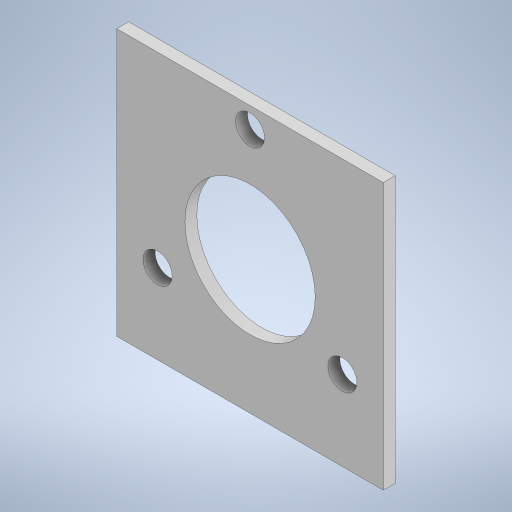
# Autodesk Inventor part: mount_v06
Saved by Autodesk Inventor 2024 (Build 280153000, 153)
## iProperties
Created: 2025-07-16
Part Number: mount_v06
Material: Generic
Document SubType Name: Modeling
Designer: Akramilab
Density: 1 g/cm^3
Appearance: Default
Author: Akramilab
Autodesk Inventor part; units mm, degrees
ref_plane "YZ Plane" through (0, 0, 0) normal (1, 0, 0) x (0, 1, 0)
ref_plane "XZ Plane" through (0, 0, 0) normal (0, 1, 0) x (-1, 0, 0)
ref_plane "XY Plane" through (0, 0, 0) normal (0, 0, 1) x (1, 0, 0)
sketch "Sketch1" plane through (0, 0, 0) normal (0, 0, 1) x (1, 0, 0)
  line L0 (-22.5, -22.5) -> (22.5, -22.5)
  line L1 (22.5, -22.5) -> (22.5, 22.5)
  line L2 (22.5, 22.5) -> (-22.5, 22.5)
  line L3 (-22.5, 22.5) -> (-22.5, -22.5)
  line L4 (-22.5, -22.5) -> (22.5, 22.5) construction
  line L5 (22.5, -22.5) -> (-22.5, 22.5) construction
  circle A0 centre (0, 0) radius 11
  line L6 (0, 0) -> (0, 19)
  line L7 (0, 0) -> (15.6, -9.0067)
  line L8 (0, 0) -> (-15.6, -9.0067)
  circle A1 centre (0, 19) radius 2.45
  circle A2 centre (15.6, -9.0067) radius 2.45
  circle A3 centre (-15.6, -9.0067) radius 2.45
  point P0 (22.5, -11.0947)
  point P1 (-22.5, -11.0947)
  dimension "d0" = 45
  dimension "d1" = 45
  dimension "d2" = 22
  dimension "d3" = 19
  dimension "d4" = 15.6
  dimension "d5" = 120
  dimension "d6" = 15.6
  dimension "d7" = 120
  dimension "d8" = 4.9
  dimension "d9" = 4.9
  dimension "d10" = 4.9
  constraints: 18 end point, 4 centre point, 4 coincident, 2 midpoint, 2 parallel, 2 point on line, 1 horizontal, 1 perpendicular, 1 vertical
  measures "d0" distance of L2.end L1.end
  measures "d1" distance of L1.end L0.end
  measures "d2" diameter of A0
  measures "d3" distance of L6.start L6.end
  measures "d4" horizontal distance of L7.start L7.end
  measures "d5" angle of L7 L6
  measures "d6" horizontal distance of L7.start L8.end
  measures "d7" angle of L8 L7
  measures "d8" diameter of A1
  measures "d9" diameter of A2
  measures "d10" diameter of A3
extrude "Extrusion2" add sketch "Sketch1" along normal blind 2
equation "\"d1\" = d0"
equation "\"d4\" = d6"
equation "\"d7\" = d5"
equation "\"d9\" = d8"
equation "\"d10\" = d8"
body "Solid2"
